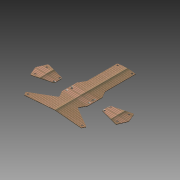
# Autodesk Inventor part: Veroboard Bottom Plate
Saved by Autodesk Inventor 2015 (Build 190159000, 159)
## iProperties
Created: 2015-10-10
Part Number: Veroboard Bottom Plate
Material: Veroboard
Document SubType Name: Modeling
Designer: James
Density: 1 g/cm^3
Appearance: Generic
Mass: 9.80683 g
Surface Area: 205.36 cm^2
Volume: 9.80683 cm^3
Author: James
Autodesk Inventor part; units mm, degrees
ref_plane "YZ Plane" through (0, 0, 0) normal (1, 0, 0) x (0, 1, 0)
ref_plane "XZ Plane" through (0, 0, 0) normal (0, 1, 0) x (-1, 0, 0)
ref_plane "XY Plane" through (0, 0, 0) normal (0, 0, 1) x (1, 0, 0)
sketch "Sketch1" plane through (0, 0, 0) normal (0, 1, 0) x (-1, 0, 0)
  line L0 (-18.4808, -28.5263) -> (-18.4808, -88.5379)
  line L1 (25.7128, 15.4641) -> (19.4808, 26.2583)
  arc A0 (20.2128, 28.9904) -> (19.4808, 26.2583) centre (21.2128, 27.2583) ccw
  arc A1 (-60.782, 54.7224) -> (-60.05, 51.9904) centre (-59.05, 53.7224) ccw
  line L2 (-20.2128, 28.9904) -> (-60.05, 51.9904)
  arc A2 (60.05, 51.9904) -> (60.782, 54.7224) centre (59.05, 53.7224) ccw
  line L3 (20.2128, 28.9904) -> (60.05, 51.9904)
  arc A3 (-85.4804, 17.9488) -> (-87.8378, 16.8012) centre (-85.998, 16.0169) ccw
  arc A4 (-94.6657, 0.7843) -> (-94.6657, -0.7843) centre (-92.8259, 0) ccw
  arc A5 (-87.8378, -16.8012) -> (-85.4804, -17.9488) centre (-85.998, -16.0169) ccw
  line L4 (-94.6657, -0.7843) -> (-87.8378, -16.8012)
  line L5 (-94.6657, 0.7843) -> (-87.8378, 16.8012)
  arc A6 (48.5201, -6.5107) -> (50.0024, -8.4425) centre (50.5201, -6.5107) ccw
  line L6 (48.5201, -6.5107) -> (48.5201, 6.5107)
  arc A7 (50.0024, 8.4425) -> (48.5201, 6.5107) centre (50.5201, 6.5107) ccw
  line L7 (85.4804, 17.9488) -> (50.0024, 8.4425)
  line L8 (85.4804, -17.9488) -> (50.0024, -8.4425)
  arc A8 (87.8378, 16.8012) -> (85.4804, 17.9488) centre (85.998, 16.0169) ccw
  line L9 (94.6657, 0.7843) -> (87.8378, 16.8012)
  line L10 (-18.4808, -88.5379) -> (-18.4808, -91.8911)
  line L11 (18.4808, -88.5379) -> (18.4808, -91.8911)
  line L12 (18.4808, -28.5263) -> (18.4808, -88.5379)
  line L13 (-25.7128, -15.4641) -> (-18.7487, -27.5263)
  arc A9 (-25.9808, -14.4641) -> (-25.7128, -15.4641) centre (-23.9808, -14.4641) ccw
  arc A10 (-18.4808, -28.5263) -> (-18.7487, -27.5263) centre (-20.4808, -28.5263) ccw
  line L14 (-85.4804, 17.9488) -> (-50.0024, 8.4425)
  line L15 (-85.4804, -17.9488) -> (-50.0024, -8.4425)
  line L16 (25.7128, -15.4641) -> (18.7487, -27.5263)
  arc A11 (25.7128, -15.4641) -> (25.9808, -14.4641) centre (23.9808, -14.4641) ccw
  arc A12 (18.7487, -27.5263) -> (18.4808, -28.5263) centre (20.4808, -28.5263) ccw
  arc A13 (25.9808, 14.4641) -> (25.7128, 15.4641) centre (23.9808, 14.4641) ccw
  line L17 (25.9808, 14.4641) -> (25.9808, -14.4641)
  arc A14 (85.4804, -17.9488) -> (87.8378, -16.8012) centre (85.998, -16.0169) ccw
  arc A15 (94.6657, -0.7843) -> (94.6657, 0.7843) centre (92.8259, 0) ccw
  line L18 (94.6657, -0.7843) -> (87.8378, -16.8012)
  line L19 (-25.9808, 14.4641) -> (-25.9808, -14.4641)
  line L20 (-25.7128, 15.4641) -> (-19.4808, 26.2583)
  arc A16 (-25.7128, 15.4641) -> (-25.9808, 14.4641) centre (-23.9808, 14.4641) ccw
  arc A17 (-19.4808, 26.2583) -> (-20.2128, 28.9904) centre (-21.2128, 27.2583) ccw
  arc A18 (-50.0024, -8.4425) -> (-48.5201, -6.5107) centre (-50.5201, -6.5107) ccw
  line L21 (-48.5201, -6.5107) -> (-48.5201, 6.5107)
  arc A19 (-48.5201, 6.5107) -> (-50.0024, 8.4425) centre (-50.5201, 6.5107) ccw
  arc A20 (-18.4808, -91.8911) -> (18.4808, -91.8911) centre (0, 0) ccw
  line L22 (-18.4808, -91.8911) -> (-18.4808, -28.5263)
  line L23 (-18.7487, -27.5263) -> (-25.7128, -15.4641)
  line L24 (-25.9808, -14.4641) -> (-25.9808, 14.4641)
  line L25 (-25.7128, 15.4641) -> (-19.4808, 26.2583)
  line L26 (-20.2128, 28.9904) -> (-60.05, 51.9904)
  line L27 (60.05, 51.9904) -> (20.2128, 28.9904)
  line L28 (19.4808, 26.2583) -> (25.7128, 15.4641)
  line L29 (25.9808, 14.4641) -> (25.9808, -14.4641)
  line L30 (25.7128, -15.4641) -> (18.7487, -27.5263)
  line L31 (18.4808, -28.5263) -> (18.4808, -91.8911)
  arc A21 (-18.4808, -28.5263) -> (-18.7487, -27.5263) centre (-20.4808, -28.5263) ccw
  arc A22 (-25.9808, -14.4641) -> (-25.7128, -15.4641) centre (-23.9808, -14.4641) ccw
  arc A23 (-25.7128, 15.4641) -> (-25.9808, 14.4641) centre (-23.9808, 14.4641) ccw
  arc A24 (-19.4808, 26.2583) -> (-20.2128, 28.9904) centre (-21.2128, 27.2583) ccw
  arc A25 (-60.782, 54.7224) -> (-60.05, 51.9904) centre (-59.05, 53.7224) ccw
  arc A26 (60.05, 51.9904) -> (60.782, 54.7224) centre (59.05, 53.7224) ccw
  arc A27 (20.2128, 28.9904) -> (19.4808, 26.2583) centre (21.2128, 27.2583) ccw
  arc A28 (25.9808, 14.4641) -> (25.7128, 15.4641) centre (23.9808, 14.4641) ccw
  arc A29 (25.7128, -15.4641) -> (25.9808, -14.4641) centre (23.9808, -14.4641) ccw
  arc A30 (18.7487, -27.5263) -> (18.4808, -28.5263) centre (20.4808, -28.5263) ccw
  line L32 (-50.0024, -8.4425) -> (-85.4804, -17.9488)
  line L33 (-87.8378, -16.8012) -> (-94.6657, -0.7843)
  line L34 (-94.6657, 0.7843) -> (-87.8378, 16.8012)
  line L35 (-85.4804, 17.9488) -> (-50.0024, 8.4425)
  line L36 (-48.5201, 6.5107) -> (-48.5201, -6.5107)
  arc A31 (-87.8378, -16.8012) -> (-85.4804, -17.9488) centre (-85.998, -16.0169) ccw
  arc A32 (-94.6657, 0.7843) -> (-94.6657, -0.7843) centre (-92.8259, 0) ccw
  arc A33 (-85.4804, 17.9488) -> (-87.8378, 16.8012) centre (-85.998, 16.0169) ccw
  arc A34 (-48.5201, 6.5107) -> (-50.0024, 8.4425) centre (-50.5201, 6.5107) ccw
  arc A35 (-50.0024, -8.4425) -> (-48.5201, -6.5107) centre (-50.5201, -6.5107) ccw
  arc A36 (48.5201, -6.5107) -> (50.0024, -8.4425) centre (50.5201, -6.5107) ccw
  arc A37 (50.0024, 8.4425) -> (48.5201, 6.5107) centre (50.5201, 6.5107) ccw
  arc A38 (85.4804, -17.9488) -> (87.8378, -16.8012) centre (85.998, -16.0169) ccw
  arc A39 (94.6657, -0.7843) -> (94.6657, 0.7843) centre (92.8259, 0) ccw
  arc A40 (87.8378, 16.8012) -> (85.4804, 17.9488) centre (85.998, 16.0169) ccw
  line L37 (87.8378, -16.8012) -> (94.6657, -0.7843)
  line L38 (94.6657, 0.7843) -> (87.8378, 16.8012)
  line L39 (85.4804, 17.9488) -> (50.0024, 8.4425)
  line L40 (48.5201, 6.5107) -> (48.5201, -6.5107)
  line L41 (50.0024, -8.4425) -> (85.4804, -17.9488)
  line L42 (19.4808, -26.2583) -> (25.7128, -15.4641)
  arc A41 (25.7128, -15.4641) -> (25.9808, -14.4641) centre (23.9808, -14.4641) ccw
  line L43 (25.9808, -14.4641) -> (25.9808, 14.4641)
  arc A42 (25.9808, 14.4641) -> (25.7128, 15.4641) centre (23.9808, 14.4641) ccw
  arc A43 (-25.7128, 15.4641) -> (-25.9808, 14.4641) centre (-23.9808, 14.4641) ccw
  line L44 (-25.9808, 14.4641) -> (-25.9808, -14.4641)
  arc A44 (-25.9808, -14.4641) -> (-25.7128, -15.4641) centre (-23.9808, -14.4641) ccw
  line L45 (-25.7128, -15.4641) -> (-19.4808, -26.2583)
  line L46 (-50.0024, 8.4425) -> (-85.4804, 17.9488)
  arc A45 (-85.4804, 17.9488) -> (-87.8378, 16.8012) centre (-85.998, 16.0169) ccw
  line L47 (-87.8378, 16.8012) -> (-94.6657, 0.7843)
  arc A46 (-94.6657, 0.7843) -> (-94.6657, -0.7843) centre (-92.8259, 0) ccw
  line L48 (-94.6657, -0.7843) -> (-87.8378, -16.8012)
  arc A47 (-87.8378, -16.8012) -> (-85.4804, -17.9488) centre (-85.998, -16.0169) ccw
  line L49 (-85.4804, -17.9488) -> (-50.0024, -8.4425)
  arc A48 (-50.0024, -8.4425) -> (-48.5201, -6.5107) centre (-50.5201, -6.5107) ccw
  line L50 (-48.5201, -6.5107) -> (-48.5201, 6.5107)
  arc A49 (-48.5201, 6.5107) -> (-50.0024, 8.4425) centre (-50.5201, 6.5107) ccw
  arc A50 (85.4804, -17.9488) -> (87.8378, -16.8012) centre (85.998, -16.0169) ccw
  line L51 (87.8378, -16.8012) -> (94.6657, -0.7843)
  arc A51 (94.6657, -0.7843) -> (94.6657, 0.7843) centre (92.8259, 0) ccw
  line L52 (94.6657, 0.7843) -> (87.8378, 16.8012)
  arc A52 (87.8378, 16.8012) -> (85.4804, 17.9488) centre (85.998, 16.0169) ccw
  line L53 (85.4804, 17.9488) -> (50.0024, 8.4425)
  arc A53 (50.0024, 8.4425) -> (48.5201, 6.5107) centre (50.5201, 6.5107) ccw
  line L54 (48.5201, 6.5107) -> (48.5201, -6.5107)
  arc A54 (48.5201, -6.5107) -> (50.0024, -8.4425) centre (50.5201, -6.5107) ccw
  line L55 (50.0024, -8.4425) -> (85.4804, -17.9488)
  line L56 (57.782, 59.9186) -> (0, 55)
  line L57 (-57.782, 59.9186) -> (0, 55)
  line L58 (-57.782, 59.9186) -> (-60.782, 54.7224)
  line L59 (57.782, 59.9186) -> (60.782, 54.7224)
  line L60 (18.4808, -91.8911) -> (18.4808, -88.5379)
  line L61 (18.4808, -91.8911) -> (18.4808, -89.8911)
  circle A55 centre (-54.9519, 54.8205) radius 1.65
  circle A56 centre (54.9519, 54.8205) radius 1.65
  circle A57 centre (-20.9808, 0) radius 1.65
  circle A58 centre (20.9808, 0) radius 1.65
  circle A59 centre (-14.6505, -86.7861) radius 1.65
  circle A60 centre (14.6505, -86.7861) radius 1.65
  circle A61 centre (51.6401, 6.133) radius 1.65
  circle A62 centre (51.6401, -6.133) radius 1.65
  circle A63 centre (83.498, 11.6868) radius 1.65
  circle A64 centre (83.498, -11.6868) radius 1.65
  circle A65 centre (-51.6401, 6.133) radius 1.65
  circle A66 centre (-51.6401, -6.133) radius 1.65
  circle A67 centre (-83.498, 11.6868) radius 1.65
  circle A68 centre (-83.498, -11.6868) radius 1.65
  dimension "d19" = 2
  constraints: 124 end point, 110 point on circle, 69 centre point, 20 coincident, 18 collinear, 7 tangent, 3 vertical, 1 perpendicular, 1 point on line
  measures "d19" distance of L31.end L61.end
ref_plane "Work Plane2" through (0, 1, 0) normal (0, 1, 0) x (1, 0, 0)
extrude "Extrusion5" add sketch "Sketch1" along normal blind 1
sketch "Sketch2" plane through (0, 1, 0) normal (0, 1, 0) x (1, 0, 0)
  circle A0 centre (-14.6505, 21.7861) radius 1.25 projected
  circle A1 centre (-14.6505, 87.3566) radius 1.25 projected
  circle A2 centre (-44.6505, -51.9904) radius 1.25 projected
  circle A3 centre (14.6505, 21.7861) radius 1.25 projected
  circle A4 centre (44.6505, -51.9904) radius 1.25 projected
  circle A5 centre (14.6505, -51.9904) radius 1.25 projected
  circle A6 centre (14.6505, -18.2139) radius 1.25 projected
  circle A7 centre (-14.6505, -51.9904) radius 1.25 projected
  circle A8 centre (14.6505, 71.7861) radius 1.25 projected
  circle A9 centre (-14.6505, 71.7861) radius 1.25 projected
  line L0 (60.05, -51.9904) -> (20.2128, -28.9904) projected
  arc A10 (19.4808, -26.2583) -> (20.2128, -28.9904) centre (21.2128, -27.2583) ccw projected
  line L1 (19.4808, -26.2583) -> (25.7128, -15.4641) projected
  arc A11 (25.7128, -15.4641) -> (25.9808, -14.4641) centre (23.9808, -14.4641) ccw projected
  line L2 (25.9808, -14.4641) -> (25.9808, 14.4641) projected
  arc A12 (25.9808, 14.4641) -> (25.7128, 15.4641) centre (23.9808, 14.4641) ccw projected
  line L3 (25.7128, 15.4641) -> (18.7487, 27.5263) projected
  arc A13 (18.4808, 28.5263) -> (18.7487, 27.5263) centre (20.4808, 28.5263) ccw projected
  line L4 (18.4808, 28.5263) -> (18.4808, 91.8911) projected
  arc A14 (18.4808, 91.8911) -> (-18.4808, 91.8911) centre (0, 0) ccw projected
  line L5 (-18.4808, 91.8911) -> (-18.4808, 28.5263) projected
  arc A15 (-18.7487, 27.5263) -> (-18.4808, 28.5263) centre (-20.4808, 28.5263) ccw projected
  line L6 (-18.7487, 27.5263) -> (-25.7128, 15.4641) projected
  arc A16 (-25.7128, 15.4641) -> (-25.9808, 14.4641) centre (-23.9808, 14.4641) ccw projected
  line L7 (-25.9808, 14.4641) -> (-25.9808, -14.4641) projected
  arc A17 (-25.9808, -14.4641) -> (-25.7128, -15.4641) centre (-23.9808, -14.4641) ccw projected
  line L8 (-25.7128, -15.4641) -> (-19.4808, -26.2583) projected
  arc A18 (-20.2128, -28.9904) -> (-19.4808, -26.2583) centre (-21.2128, -27.2583) ccw projected
  line L9 (-20.2128, -28.9904) -> (-60.05, -51.9904) projected
  arc A19 (-60.05, -51.9904) -> (-60.782, -54.7224) centre (-59.05, -53.7224) ccw projected
  line L10 (-60.782, -54.7224) -> (-57.782, -59.9186) projected
  line L11 (-57.782, -59.9186) -> (0, -55) projected
  line L12 (0, -55) -> (57.782, -59.9186) projected
  line L13 (57.782, -59.9186) -> (60.782, -54.7224) projected
  arc A20 (60.782, -54.7224) -> (60.05, -51.9904) centre (59.05, -53.7224) ccw projected
  line L14 (-18.4808, 91.8911) -> (-18.4808, 89.8911)
  line L15 (-18.4808, 91.8911) -> (-18.4808, 28.5263) projected
  line L16 (18.4808, 91.8911) -> (18.4808, 89.8911)
  line L17 (18.4808, 28.5263) -> (18.4808, 91.8911) projected
  arc A21 (18.4808, 91.8911) -> (-18.4808, 91.8911) centre (0, 0) ccw
  arc A22 (18.4808, 89.8911) -> (-18.4808, 89.8911) centre (0, 0) ccw
  dimension "d20" = 2
  constraints: 4 end point, 4 point on circle, 2 centre point, 2 coincident, 2 point on line
  measures "d20" distance of L5.start L14.end
extrude "Extrusion2" cut sketch "Sketch2" against normal blind 1 contours A22 L5 A14 L4
body "Solid1"
